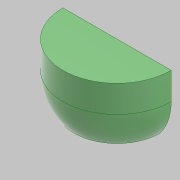
# Autodesk Inventor part: 본체
Saved by Autodesk Inventor 2020 (Build 240168000, 168)
## iProperties
Created: 2020-05-03
Part Number: 본체
Material: 일반
Document SubType Name: Modeling
Designer: sbahn
Density: 1 g/cm^3
Appearance: 매끄러움 - 짙은 산림 녹색
Author: sbahn
Autodesk Inventor part; units mm, degrees
(part 1 of 2)
ref_plane "XZ Plane" through (0, 0, 0) normal (0, 1, 0) x (-1, 0, 0)
ref_plane "XY Plane" through (0, 0, 0) normal (0, 0, 1) x (1, 0, 0)
sketch "스케치1" plane through (0, 0, 0) normal (0, 1, 0) x (-1, 0, 0)
  line L0 (-14.5321, -10.5819) -> (-29.968, -35.283)
  arc A0 (-38.4205, -39.9689) -> (-29.968, -35.283) centre (-38.422, -30) ccw
  line L1 (-38.4205, -39.9689) -> (-120.878, -39.9798)
  line L2 (-120.8795, 40) -> (-38.422, 40)
  arc A1 (-29.942, 35.3) -> (-38.422, 40) centre (-38.422, 30) ccw
  line L3 (-29.942, 35.3) -> (-14.5328, 10.583)
  line L4 (-18.7445, -7.95) -> (-34.182, -32.65)
  arc A2 (-38.422, -35) -> (-34.182, -32.65) centre (-38.422, -30) ccw
  line L5 (-38.422, -35) -> (-120.8795, -35)
  line L6 (-120.8795, 35) -> (-38.422, 35)
  arc A3 (-34.182, 32.65) -> (-38.422, 35) centre (-38.422, 30) ccw
  line L7 (-34.182, 32.65) -> (-18.7445, 7.95)
  line L8 (-133.9879, -34.9502) -> (-133.9879, -34.9502)
  line L9 (0, 0) -> (-214.2408, 0)
  line L10 (-97.3795, -37.5) -> (-100.3795, -37.5)
  line L11 (-104.8795, -3.3) -> (-104.8795, -27.5)
  line L12 (-66.878, -39.9727) -> (-66.8787, -35)
  line L13 (-62.878, -39.9722) -> (-62.8787, -35)
  line L14 (-64.8795, -35) -> (-64.8795, -34)
  line L15 (-80.8795, -35) -> (-80.8795, -34)
  line L16 (-78.8787, -35) -> (-78.878, -39.9743)
  line L17 (-59.8795, -39.9718) -> (-59.8795, -48)
  line L18 (-85.8795, -48) -> (-85.8795, -39.9752)
  line L19 (-67.8795, -39.9728) -> (-67.8795, -48)
  line L20 (-73.8795, -29) -> (-73.8795, -83)
  line L21 (-71.8795, -83) -> (-71.8795, -29)
  line L22 (-85.8795, -48) -> (-59.8795, -48)
  line L23 (-77.8795, -48) -> (-77.8795, -39.9741)
  line L24 (-87.7712, -44) -> (-71.8795, -44)
  line L25 (-85.8795, -45.5) -> (-77.8795, -45.5)
  line L26 (-85.8795, -42.5) -> (-77.8795, -42.5)
  line L27 (-77.8795, -42.5) -> (-76.2373, -44)
  line L28 (-76.2373, -44) -> (-77.8795, -45.5)
  line L29 (-72.8795, -48) -> (-55.3795, -48)
  line L30 (-90.3795, -53) -> (-90.3795, -48)
  line L31 (-127.8795, -53) -> (-127.8795, -89)
  line L32 (-127.8795, -89) -> (-17.8795, -89)
  line L33 (-17.8795, -89) -> (-17.8795, -53)
  line L34 (-17.8795, -53) -> (-127.8795, -53)
  line L35 (-126.8795, -54) -> (-18.8795, -54)
  line L36 (-18.8795, -54) -> (-18.8795, -88)
  line L37 (-18.8795, -88) -> (-126.8795, -88)
  line L38 (-126.8795, -88) -> (-126.8795, -54)
  line L39 (-55.3795, -59) -> (-90.3795, -59)
  line L40 (-90.3795, -54) -> (-90.3795, -59)
  line L41 (-71.8795, -48) -> (-71.8795, -59)
  line L42 (-73.8795, -48) -> (-73.8795, -59)
  line L43 (-85.8795, -48) -> (-90.3795, -48)
  line L44 (-88.1295, -46.2635) -> (-88.1295, -60.7681)
  line L45 (-57.6295, -46.0218) -> (-57.6295, -60.2242)
  line L46 (-87.1295, -49.1111) -> (-85.8795, -48)
  line L47 (-89.1295, -49.1111) -> (-90.3795, -48)
  line L48 (-89.1295, -49.1111) -> (-89.1295, -59)
  line L49 (-87.1295, -49.1111) -> (-87.1295, -59)
  line L50 (-87.1295, -49.1111) -> (-89.1295, -49.1111)
  line L51 (-55.3795, -53) -> (-55.3795, -48)
  line L52 (-55.3795, -54) -> (-55.3795, -59)
  line L53 (-58.6295, -49.1111) -> (-59.8795, -48)
  line L54 (-56.6295, -49.1111) -> (-55.3795, -48)
  line L55 (-56.6295, -49.1111) -> (-56.6295, -59)
  line L56 (-58.6295, -49.1111) -> (-58.6295, -59)
  line L57 (-58.6295, -49.1111) -> (-56.6295, -49.1111)
  line L58 (-8.3175, -71) -> (-138.1557, -71)
  line L59 (-90.3795, -94) -> (-78.8795, -94)
  line L60 (-66.8795, -94) -> (-55.3795, -94)
  line L61 (-90.3795, -89) -> (-90.3795, -94)
  line L62 (-55.3795, -83) -> (-90.3795, -83)
  line L63 (-90.3795, -88) -> (-90.3795, -83)
  line L64 (-71.8795, -92) -> (-71.8795, -83)
  line L65 (-73.8795, -92) -> (-73.8795, -83)
  line L66 (-88.1295, -95.7365) -> (-88.1295, -81.2319)
  line L67 (-57.6295, -95.9782) -> (-57.6295, -81.7758)
  line L68 (-87.1295, -92.8889) -> (-85.8795, -94)
  line L69 (-89.1295, -92.8889) -> (-90.3795, -94)
  line L70 (-89.1295, -92.8889) -> (-89.1295, -83)
  line L71 (-87.1295, -92.8889) -> (-87.1295, -83)
  line L72 (-87.1295, -92.8889) -> (-89.1295, -92.8889)
  line L73 (-55.3795, -89) -> (-55.3795, -94)
  line L74 (-55.3795, -88) -> (-55.3795, -83)
  line L75 (-58.6295, -92.8889) -> (-59.8795, -94)
  line L76 (-56.6295, -92.8889) -> (-55.3795, -94)
  line L77 (-56.6295, -92.8889) -> (-56.6295, -83)
  line L78 (-58.6295, -92.8889) -> (-58.6295, -83)
  line L79 (-58.6295, -92.8889) -> (-56.6295, -92.8889)
  line L80 (-74.8795, -71) -> (-70.8795, -71)
  line L81 (-71.8795, -83) -> (-71.8795, -59)
  line L82 (-73.8795, -59) -> (-73.8795, -83)
  line L83 (-72.8795, -59) -> (-64.8795, -59)
  line L84 (-64.8795, -59) -> (-70.8795, -71)
  line L85 (-72.8795, -59) -> (-80.8795, -59)
  line L86 (-80.8795, -59) -> (-74.8795, -71)
  line L87 (-72.8795, -83) -> (-80.8795, -83)
  line L88 (-80.8795, -83) -> (-74.8795, -71)
  line L89 (-72.8795, -83) -> (-64.8795, -83)
  line L90 (-64.8795, -83) -> (-70.8795, -71)
  line L91 (-66.8795, 40) -> (-66.8795, 35)
  line L92 (-62.8795, 40) -> (-62.8795, 35)
  line L93 (-64.8795, 35) -> (-64.8795, 34)
  line L94 (-80.8795, 35) -> (-80.8795, 34)
  line L95 (-78.8795, 35) -> (-78.8795, 40)
  line L96 (-59.8795, 40) -> (-59.8795, 48)
  line L97 (-85.8795, 48) -> (-85.8795, 40)
  line L98 (-67.8795, 40) -> (-67.8795, 48)
  line L99 (-73.8795, 29) -> (-73.8795, 48)
  line L100 (-71.8795, 48) -> (-71.8795, 29)
  line L101 (-85.8795, 48) -> (-59.8795, 48)
  line L102 (-77.8795, 48) -> (-77.8795, 40)
  line L103 (-87.7712, 44) -> (-71.8795, 44)
  line L104 (-85.8795, 45.5) -> (-77.8795, 45.5)
  line L105 (-85.8795, 42.5) -> (-77.8795, 42.5)
  line L106 (-77.8795, 42.5) -> (-76.2373, 44)
  line L107 (-76.2373, 44) -> (-77.8795, 45.5)
  line L108 (-72.8795, 48) -> (-55.3795, 48)
  line L109 (-90.3795, 53) -> (-90.3795, 48)
  line L110 (-127.8795, 53) -> (-127.8795, 89)
  line L111 (-127.8795, 89) -> (-17.8795, 89)
  line L112 (-17.8795, 89) -> (-17.8795, 53)
  line L113 (-17.8795, 53) -> (-127.8795, 53)
  line L114 (-126.8795, 54) -> (-18.8795, 54)
  line L115 (-18.8795, 54) -> (-18.8795, 88)
  line L116 (-18.8795, 88) -> (-126.8795, 88)
  line L117 (-126.8795, 88) -> (-126.8795, 54)
  line L118 (-55.3795, 59) -> (-90.3795, 59)
  line L119 (-90.3795, 54) -> (-90.3795, 59)
  line L120 (-71.8795, 48) -> (-71.8795, 59)
  line L121 (-73.8795, 48) -> (-73.8795, 59)
  line L122 (-85.8795, 48) -> (-90.3795, 48)
  line L123 (-88.1295, 46.2635) -> (-88.1295, 60.7681)
  line L124 (-57.6295, 46.0218) -> (-57.6295, 60.2242)
  line L125 (-87.1295, 49.1111) -> (-85.8795, 48)
  line L126 (-89.1295, 49.1111) -> (-90.3795, 48)
  line L127 (-89.1295, 49.1111) -> (-89.1295, 59)
  line L128 (-87.1295, 49.1111) -> (-87.1295, 59)
  line L129 (-87.1295, 49.1111) -> (-89.1295, 49.1111)
  line L130 (-55.3795, 53) -> (-55.3795, 48)
  line L131 (-55.3795, 54) -> (-55.3795, 59)
  line L132 (-58.6295, 49.1111) -> (-59.8795, 48)
  line L133 (-56.6295, 49.1111) -> (-55.3795, 48)
  line L134 (-56.6295, 49.1111) -> (-56.6295, 59)
  line L135 (-58.6295, 49.1111) -> (-58.6295, 59)
  line L136 (-58.6295, 49.1111) -> (-56.6295, 49.1111)
  line L137 (-8.3175, 71) -> (-138.1557, 71)
  line L138 (-90.3795, 94) -> (-78.8795, 94)
  line L139 (-66.8795, 94) -> (-55.3795, 94)
  line L140 (-55.3795, 94) -> (-55.3795, 89)
  line L141 (-90.3795, 89) -> (-90.3795, 94)
  line L142 (-55.3795, 88) -> (-55.3795, 83)
  line L143 (-55.3795, 83) -> (-90.3795, 83)
  line L144 (-90.3795, 88) -> (-90.3795, 83)
  line L145 (-71.8795, 92) -> (-71.8795, 48)
  line L146 (-73.8795, 92) -> (-73.8795, 48)
  line L147 (-88.1295, 95.7365) -> (-88.1295, 81.2319)
  line L148 (-57.6295, 95.9782) -> (-57.6295, 81.7758)
  line L149 (-87.1295, 92.8889) -> (-85.8795, 94)
  line L150 (-89.1295, 92.8889) -> (-90.3795, 94)
  line L151 (-89.1295, 92.8889) -> (-89.1295, 83)
  line L152 (-87.1295, 92.8889) -> (-87.1295, 83)
  line L153 (-87.1295, 92.8889) -> (-89.1295, 92.8889)
  line L154 (-58.6295, 92.8889) -> (-59.8795, 94)
  line L155 (-56.6295, 92.8889) -> (-55.3795, 94)
  line L156 (-56.6295, 92.8889) -> (-56.6295, 83)
  line L157 (-58.6295, 92.8889) -> (-58.6295, 83)
  line L158 (-58.6295, 92.8889) -> (-56.6295, 92.8889)
  line L159 (-74.8795, 71) -> (-70.8795, 71)
  line L160 (-71.8795, 83) -> (-71.8795, 59)
  line L161 (-73.8795, 59) -> (-73.8795, 83)
  line L162 (-72.8795, 59) -> (-64.8795, 59)
  line L163 (-64.8795, 59) -> (-70.8795, 71)
  line L164 (-72.8795, 59) -> (-80.8795, 59)
  line L165 (-80.8795, 59) -> (-74.8795, 71)
  line L166 (-72.8795, 83) -> (-80.8795, 83)
  line L167 (-80.8795, 83) -> (-74.8795, 71)
  line L168 (-72.8795, 83) -> (-64.8795, 83)
  line L169 (-64.8795, 83) -> (-70.8795, 71)
  line L170 (-72.8795, -104.0341) -> (-72.8795, 102.0223)
  line L171 (-85.8795, -28) -> (-85.8795, -35)
  line L172 (-87.8795, -29) -> (-87.8795, -34)
  line L173 (-88.3795, -29) -> (-88.3795, -34)
  line L174 (-83.3795, -29) -> (-83.3795, -34)
  line L175 (-59.8795, -28) -> (-59.8795, -35)
  line L176 (-57.8795, -29) -> (-57.8795, -34)
  line L177 (-62.3795, -29) -> (-62.3795, -34)
  line L178 (-57.8795, -34) -> (-113.8795, -34)
  line L179 (-57.8795, -29) -> (-113.8795, -29)
  line L180 (-111.8795, -28) -> (-111.8795, -35)
  line L181 (-113.8795, -29) -> (-113.8795, -34)
  line L182 (-109.3795, -29) -> (-109.3795, -34)
  line L183 (-98.8795, -45.3206) -> (-98.8795, 49.0244)
  line L184 (-82.8795, 35) -> (-82.8795, 40)
  line L185 (-100.8795, -27.5) -> (-100.8795, -28.3)
  line L186 (-100.8795, -28.3) -> (-96.8795, -28.3)
  line L187 (-96.8795, -28.3) -> (-96.8795, -27.5)
  line L188 (-100.3795, -38) -> (-97.3795, -38)
  line L189 (-109.7745, -27.5) -> (-87.8795, -27.5)
  line L190 (-97.3795, 37.5) -> (-100.3795, 37.5)
  line L191 (-104.8795, 3.3) -> (-104.8795, 27.5)
  line L192 (-111.8795, 28) -> (-111.8795, 35)
  line L193 (-113.8795, 29) -> (-113.8795, 34)
  line L194 (-109.3795, 29) -> (-109.3795, 34)
  line L195 (-100.8795, 27.5) -> (-100.8795, 28.3)
  line L196 (-100.8795, 28.3) -> (-96.8795, 28.3)
  line L197 (-96.8795, 28.3) -> (-96.8795, 27.5)
  line L198 (-100.3795, 38) -> (-100.3795, 27.5)
  line L199 (-100.3795, 38) -> (-97.3795, 38)
  line L200 (-97.3795, 38) -> (-97.3795, 27.5)
  line L201 (-109.8795, 27.5) -> (-87.8795, 27.5)
  line L202 (-87.8795, 27.5) -> (-87.8795, -27.5)
  line L203 (-109.8795, 27.5) -> (-109.8795, 9.2)
  line L204 (-109.7745, -9.2011) -> (-109.7745, -27.5)
  line L205 (-85.8795, 28) -> (-85.8795, 35)
  line L206 (-87.8795, 29) -> (-87.8795, 34)
  line L207 (-88.3795, 29) -> (-88.3795, 34)
  line L208 (-83.3795, 29) -> (-83.3795, 34)
  line L209 (-59.8795, 28) -> (-59.8795, 35)
  line L210 (-57.8795, 29) -> (-57.8795, 34)
  line L211 (-62.3795, 29) -> (-62.3795, 34)
  line L212 (-57.8795, 34) -> (-113.8795, 34)
  line L213 (-57.8795, 29) -> (-113.8795, 29)
  line L214 (-87.8795, -14.5) -> (-92.8795, -14.5)
  line L215 (-104.8795, -14.5) -> (-109.7745, -14.5)
  circle A4 centre (-90.3795, -14.5) radius 1.5
  circle A5 centre (-107.3795, -14.5) radius 1.5
  line L216 (-90.3795, -16.8389) -> (-90.3795, -12.0774)
  line L217 (-107.3795, -16.983) -> (-107.3795, -11.7622)
  line L218 (-87.8795, 14.5) -> (-92.8795, 14.5)
  line L219 (-104.8795, 14.5) -> (-109.8795, 14.5)
  circle A6 centre (-90.3795, 14.5) radius 1.5
  circle A7 centre (-107.3795, 14.5) radius 1.5
  line L220 (-90.3795, 16.8389) -> (-90.3795, 12.0774)
  line L221 (-107.3795, 16.983) -> (-107.3795, 11.7622)
  line L222 (-108.5248, -3.3) -> (-91.8795, -3.3)
  line L223 (-91.8795, -3.3) -> (-91.8795, 3.3)
  line L224 (-91.8795, 3.3) -> (-108.5248, 3.3)
  line L225 (-94.453, 3.3) -> (-94.453, 2.069)
  line L226 (-94.453, 2.069) -> (-94.1325, 2.069)
  line L227 (-94.1325, 2.069) -> (-94.1325, 3.3)
  line L228 (-103.306, 3.3) -> (-103.306, 2.069)
  line L229 (-103.306, 2.069) -> (-103.6265, 2.069)
  line L230 (-103.6265, 2.069) -> (-103.6265, 3.3)
  line L231 (-96.5487, 3.3) -> (-96.5487, 2.7093)
  line L232 (-96.5487, 2.7093) -> (-101.2104, 2.7093)
  line L233 (-101.2104, 3.3) -> (-101.2104, 2.7093)
  line L234 (-92.8795, 27.5) -> (-92.8795, 3.3)
  line L235 (-82.8787, -35) -> (-82.878, -39.9748)
  line L236 (-92.8795, -27.5) -> (-92.8795, -3.3)
  line L237 (-100.3795, -38) -> (-100.3795, -27.5)
  line L238 (-97.3795, -27.5) -> (-97.3795, -38)
  line L239 (-94.453, -3.3) -> (-94.453, -2.069)
  line L240 (-94.453, -2.069) -> (-94.1325, -2.069)
  line L241 (-94.1325, -2.069) -> (-94.1325, -3.3)
  line L242 (-103.306, -3.3) -> (-103.306, -2.069)
  line L243 (-103.306, -2.069) -> (-103.6265, -2.069)
  line L244 (-103.6265, -2.069) -> (-103.6265, -3.3)
  line L245 (-96.5487, -3.3) -> (-96.5487, -2.7093)
  line L246 (-96.5487, -2.7093) -> (-101.2104, -2.7093)
  line L247 (-101.2104, -3.3) -> (-101.2104, -2.7093)
  line L248 (-99.0407, 2.7093) -> (-99.0407, 2.0857)
  line L249 (-98.7184, 2.7093) -> (-98.7184, 2.0857)
  line L250 (-98.7184, 2.0857) -> (-99.0407, 2.0857)
  line L251 (-99.0407, -2.7093) -> (-99.0407, -2.0857)
  line L252 (-98.7184, -2.7093) -> (-98.7184, -2.0857)
  line L253 (-98.7184, -2.0857) -> (-99.0407, -2.0857)
  line L254 (-41.6795, -6) -> (-65.8795, -6)
  line L255 (-65.8795, -2) -> (-66.6795, -2)
  line L256 (-66.6795, -2) -> (-66.6795, 2)
  line L257 (-66.6795, 2) -> (-65.8795, 2)
  line L258 (-75.8795, -1.5) -> (-66.6795, -1.5)
  line L259 (-75.8795, 1.5) -> (-66.6795, 1.5)
  line L260 (-41.6795, 4.4265) -> (-40.4485, 4.4265)
  line L261 (-40.4485, 4.4265) -> (-40.4485, 4.747)
  line L262 (-40.4485, 4.747) -> (-41.6795, 4.747)
  line L263 (-41.6795, -4.4265) -> (-40.4485, -4.4265)
  line L264 (-40.4485, -4.4265) -> (-40.4485, -4.747)
  line L265 (-40.4485, -4.747) -> (-41.6795, -4.747)
  line L266 (-41.6795, 2.3309) -> (-41.0888, 2.3309)
  line L267 (-41.0888, 2.3309) -> (-41.0888, -2.3309)
  line L268 (-41.6795, -2.3309) -> (-41.0888, -2.3309)
  line L269 (-65.8795, 6) -> (-41.6795, 6)
  line L270 (-41.0888, -0.1611) -> (-40.4653, -0.1611)
  line L271 (-41.0888, 0.1611) -> (-40.4653, 0.1611)
  line L272 (-40.4653, 0.1611) -> (-40.4653, -0.1611)
  line L273 (-92.8795, -18.5) -> (-104.8795, -18.5)
  line L274 (-104.8795, 18.5) -> (-92.8795, 18.5)
  line L275 (-56.8795, 6) -> (-56.8795, -6)
  line L276 (-69.8795, 6.5) -> (-69.8795, -6.5)
  line L277 (-69.8795, -6.5) -> (-75.8795, -6.5)
  line L278 (-75.8795, -6.5) -> (-75.8795, 6.5)
  line L279 (-75.8795, 6.5) -> (-69.8795, 6.5)
  line L280 (-69.8795, 5) -> (-66.8795, 5)
  line L281 (-66.8795, 5) -> (-66.8795, -5)
  line L282 (-66.8795, -5) -> (-69.8795, -5)
  line L283 (-72.3795, 4.5493) -> (-72.3795, 1.5)
  line L284 (-72.3795, -1.5) -> (-72.3795, -4.5493)
  line L285 (-73.3795, 4.5493) -> (-73.3795, 1.5)
  line L286 (-73.3795, -1.5) -> (-73.3795, -4.5493)
  arc A8 (-70.3795, -6.5) -> (-75.3795, -6.5) centre (-72.8795, -7.0625) ccw
  arc A9 (-75.3795, 6.5) -> (-70.3795, 6.5) centre (-72.8795, 7.0625) ccw
  arc A10 (-14.5321, -10.5819) -> (-14.5328, 10.583) centre (-31.4645, 0) ccw
  arc A11 (-14.9564, -10.3174) -> (-14.9567, 10.3178) centre (-31.4645, 0) ccw
  arc A12 (-18.7445, -7.95) -> (-18.7445, 7.95) centre (-31.4645, 0) ccw
  arc A13 (-194.777, 7.282) -> (-194.7731, -7.2802) centre (-191.4606, 0.0018) ccw
  arc A14 (-120.8795, 40) -> (-125.0298, 39.0981) centre (-120.8795, 30) ccw
  arc A15 (-120.8795, 35) -> (-122.9546, 34.5491) centre (-120.8795, 30) ccw
  line L287 (-194.777, 7.282) -> (-125.0298, 39.0981)
  line L288 (-125.0298, 39.0981) -> (-194.7847, 7.2785)
  line L289 (-122.9546, 34.5491) -> (-178.5248, 9.2)
  arc A16 (-125.0008, -39.0412) -> (-120.878, -39.9798) centre (-120.7742, -30.0006) ccw
  arc A17 (-122.8496, -34.5501) -> (-120.8795, -35) centre (-120.7742, -30.0006) ccw
  line L290 (-194.7731, -7.2802) -> (-125.0008, -39.0412)
  line L291 (-125.0008, -39.0412) -> (-194.777, -7.2785)
  line L292 (-122.8496, -34.5501) -> (-178.4197, -9.2011)
  line L293 (-178.5248, 9.2) -> (-178.4197, -9.2011)
  line L294 (-180.4251, -9.2011) -> (-108.5248, -9.2011)
  line L295 (-108.5248, -9.2011) -> (-108.5248, 9.2)
  line L296 (-108.5248, 9.2) -> (-180.4251, 9.2)
  line L297 (-180.4251, -9.2011) -> (-180.4251, 9.2)
  line L298 (-41.6795, -10.5) -> (-65.8795, -10.5)
  line L299 (-65.8795, -10.5) -> (-65.8795, 10.5)
  line L300 (-65.8795, 10.5) -> (-41.6795, 10.5)
  line L301 (-41.6795, 10.5) -> (-41.6795, -10.5)
  circle A18 centre (-46.1795, -8.25) radius 1.5
  circle A19 centre (-61.3795, -8.25) radius 1.5
  circle A20 centre (-61.3795, 8.25) radius 1.5
  circle A21 centre (-46.1795, 8.25) radius 1.5
  line L302 (-43.3628, -8.25) -> (-63.8935, -8.25)
  line L303 (-43.3124, 8.25) -> (-63.843, 8.25)
  line L304 (-61.3795, -10.7982) -> (-61.3795, -5.405)
  line L305 (-46.1795, -11.0295) -> (-46.1795, -5.362)
  line L306 (-46.1795, 5.2057) -> (-46.1795, 11.2164)
  line L307 (-61.3795, 5.1324) -> (-61.3795, 11.1798)
  line L308 (-14.9564, -10.3174) -> (-14.3696, -10.3174)
  line L309 (-14.9567, 10.3178) -> (-14.3703, 10.3185)
  line L310 (-12.6257, -4.9057) -> (-17.7189, -4.9058)
  line L311 (-17.7189, -3.4079) -> (-20.9821, -3.4079)
  line L312 (-20.9821, -2.096) -> (-23.4937, -2.096)
  line L313 (-23.4937, -7.0903) -> (-24.761, -7.0903)
  line L314 (-12.6259, 4.9063) -> (-17.719, 4.9063)
  line L315 (-17.719, 4.9063) -> (-17.7189, -4.9058)
  line L316 (-17.719, 3.4079) -> (-20.9821, 3.4079)
  line L317 (-20.9821, 3.4079) -> (-20.9821, -3.4079)
  line L318 (-20.9821, 2.096) -> (-23.4937, 2.096)
  line L319 (-23.4937, -7.0903) -> (-23.4937, 7.0903)
  line L320 (-23.4937, 7.0903) -> (-24.761, 7.0903)
  line L321 (-24.761, 7.0903) -> (-24.761, -7.0903)
  line L322 (-12.6257, -4.9057) -> (-12.6259, 4.9063)
  line L323 (-66.8795, -94) -> (-66.8795, -92)
  line L324 (-66.8795, -92) -> (-78.8795, -92)
  line L325 (-78.8795, -92) -> (-78.8795, -94)
  line L326 (-72.8795, -92) -> (-67.8795, -92)
  line L327 (-67.8795, -92) -> (-67.8795, -95)
  line L328 (-67.8795, -95) -> (-77.8795, -95)
  line L329 (-77.8795, -95) -> (-77.8795, -92)
  line L330 (-66.8795, 94) -> (-66.8795, 92)
  line L331 (-66.8795, 92) -> (-78.8795, 92)
  line L332 (-78.8795, 92) -> (-78.8795, 94)
  line L333 (-67.8795, 92) -> (-67.8795, 95)
  line L334 (-67.8795, 95) -> (-77.8795, 95)
  line L335 (-77.8795, 95) -> (-77.8795, 92)
  line L336 (-61.6632, -40) -> (-59.8795, -41.7837)
  line L337 (-63.9083, -40) -> (-59.8795, -44.0288)
  line L338 (-66.1533, -40) -> (-59.8795, -46.2738)
  line L339 (-67.8795, -40.5189) -> (-60.3984, -48)
  line L340 (-67.8795, -42.764) -> (-62.6435, -48)
  line L341 (-67.8795, -45.009) -> (-64.8885, -48)
  line L342 (-67.8795, -47.2541) -> (-67.1336, -48)
  line L343 (-79.6237, -40) -> (-77.8795, -41.7442)
  line L344 (-81.8688, -40) -> (-79.3688, -42.5)
  line L345 (-84.1139, -40) -> (-81.6139, -42.5)
  line L346 (-78.6139, -45.5) -> (-77.8795, -46.2343)
  line L347 (-85.8795, -40.4794) -> (-83.8589, -42.5)
  line L348 (-80.8589, -45.5) -> (-78.3589, -48)
  line L349 (-83.104, -45.5) -> (-80.604, -48)
  line L350 (-85.3491, -45.5) -> (-82.8491, -48)
  line L351 (-85.8795, -47.2146) -> (-85.0941, -48)
  line L352 (-69.813, 48) -> (-67.8795, 46.0665)
  line L353 (-71.8795, 47.8214) -> (-67.8795, 43.8214)
  line L354 (-74.3032, 48) -> (-73.8795, 47.5763)
  line L355 (-71.8795, 45.5763) -> (-67.8795, 41.5763)
  line L356 (-76.5482, 48) -> (-73.8795, 45.3313)
  line L357 (-62.5482, 34) -> (-62.3795, 33.8313)
  line L358 (-71.8795, 43.3313) -> (-68.5482, 40)
  line L359 (-68.5482, 40) -> (-66.8795, 38.3313)
  line L360 (-77.8795, 47.0862) -> (-74.7933, 44)
  line L361 (-64.7933, 34) -> (-62.3795, 31.5862)
  line L362 (-74.7933, 44) -> (-73.8795, 43.0862)
  line L363 (-65.7933, 35) -> (-64.8795, 34.0862)
  line L364 (-71.8795, 41.0862) -> (-70.7933, 40)
  line L365 (-70.7933, 40) -> (-66.8795, 36.0862)
  line L366 (-76.656, 43.6176) -> (-73.8795, 40.8412)
  line L367 (-67.0384, 34) -> (-62.3795, 29.3412)
  line L368 (-71.8795, 38.8412) -> (-68.0384, 35)
  line L369 (-68.0384, 35) -> (-67.0384, 34)
  line L370 (-77.8293, 42.5459) -> (-75.2834, 40)
  line L371 (-69.2834, 34) -> (-64.2834, 29)
  line L372 (-75.2834, 40) -> (-73.8795, 38.5961)
  line L373 (-70.2834, 35) -> (-69.2834, 34)
  line L374 (-71.8795, 36.5961) -> (-70.2834, 35)
  line L375 (-77.8795, 40.351) -> (-77.5285, 40)
  line L376 (-71.5285, 34) -> (-66.5285, 29)
  line L377 (-77.5285, 40) -> (-73.8795, 36.351)
  line L378 (-71.8795, 34.351) -> (-71.5285, 34)
  line L379 (-78.8795, 39.106) -> (-74.7736, 35)
  line L380 (-71.8795, 32.106) -> (-68.7736, 29)
  line L381 (-74.7736, 35) -> (-73.8795, 34.106)
  line L382 (-78.8795, 36.8609) -> (-77.0186, 35)
  line L383 (-71.8795, 29.8609) -> (-71.0186, 29)
  line L384 (-77.0186, 35) -> (-76.0186, 34)
  line L385 (-76.0186, 34) -> (-73.8795, 31.8609)
  line L386 (-79.2637, 35) -> (-78.2637, 34)
  line L387 (-78.2637, 34) -> (-73.8795, 29.6158)
  line L388 (-80.8795, 34.3708) -> (-80.5088, 34)
  line L389 (-80.5088, 34) -> (-75.5088, 29)
  line L390 (-82.7538, 34) -> (-77.7538, 29)
  line L391 (-83.3795, 32.3806) -> (-79.9989, 29)
  line L392 (-83.3795, 30.1356) -> (-82.2439, 29)
  line L393 (-62.8795, -39.3331) -> (-63.5464, -40)
  line L394 (-62.8795, -37.088) -> (-65.7915, -40)
  line L395 (-63.0366, -35) -> (-66.8795, -38.843)
  line L396 (-65.2816, -35) -> (-66.8795, -36.5979)
  line L397 (-78.8795, -39.6176) -> (-79.2619, -40)
  line L398 (-78.8795, -37.3726) -> (-81.5069, -40)
  line L399 (-78.8795, -35.1275) -> (-82.8795, -39.1275)
  line L400 (-80.9971, -35) -> (-82.8795, -36.8825)
  line L401 (-62.41, -29) -> (-62.3795, -29.0305)
  line L402 (-64.6551, -29) -> (-62.3795, -31.2756)
  line L403 (-66.9002, -29) -> (-62.3795, -33.5206)
  line L404 (-69.1452, -29) -> (-64.1452, -34)
  line L405 (-71.3903, -29) -> (-66.3903, -34)
  line L406 (-66.3903, -34) -> (-65.3903, -35)
  line L407 (-71.8795, -30.7558) -> (-68.6354, -34)
  line L408 (-67.6354, -35) -> (-66.8795, -35.7558)
  line L409 (-68.6354, -34) -> (-67.6354, -35)
  line L410 (-75.8804, -29) -> (-73.8795, -31.0009)
  line L411 (-69.8804, -35) -> (-66.8795, -38.0009)
  line L412 (-71.8795, -33.0009) -> (-70.8804, -34)
  line L413 (-70.8804, -34) -> (-69.8804, -35)
  line L414 (-78.1255, -29) -> (-73.8795, -33.246)
  line L415 (-71.8795, -35.246) -> (-67.1255, -40)
  line L416 (-80.3705, -29) -> (-75.3705, -34)
  line L417 (-69.3705, -40) -> (-67.8795, -41.491)
  line L418 (-75.3705, -34) -> (-74.3705, -35)
  line L419 (-71.8795, -37.491) -> (-69.3705, -40)
  line L420 (-74.3705, -35) -> (-73.8795, -35.491)
  line L421 (-82.6156, -29) -> (-77.6156, -34)
  line L422 (-71.6156, -40) -> (-67.8795, -43.7361)
  line L423 (-77.6156, -34) -> (-76.6156, -35)
  line L424 (-71.8795, -39.7361) -> (-71.6156, -40)
  line L425 (-76.6156, -35) -> (-73.8795, -37.7361)
  line L426 (-83.3795, -30.4811) -> (-79.8607, -34)
  line L427 (-71.8795, -41.9811) -> (-67.8795, -45.9811)
  line L428 (-79.8607, -34) -> (-78.8607, -35)
  line L429 (-78.8607, -35) -> (-73.8795, -39.9811)
  line L430 (-83.3795, -32.7262) -> (-82.1057, -34)
  line L431 (-71.8795, -44.2262) -> (-68.1057, -48)
  line L432 (-78.8795, -37.2262) -> (-76.1057, -40)
  line L433 (-76.1057, -40) -> (-73.8795, -42.2262)
  line L434 (-78.8795, -39.4713) -> (-78.3508, -40)
  line L435 (-71.8795, -46.4713) -> (-70.3508, -48)
  line L436 (-77.8795, -40.4713) -> (-74.3508, -44)
  line L437 (-74.3508, -44) -> (-73.8795, -44.4713)
  line L438 (-76.4247, -44.1712) -> (-73.8795, -46.7163)
  line L439 (-77.598, -45.2429) -> (-74.8409, -48)
  line L440 (-77.8795, -47.2065) -> (-77.086, -48)
  line L441 (-56.6295, -54.014) -> (-55.3795, -55.264)
  line L442 (-58.8885, -54) -> (-58.6295, -54.259)
  line L443 (-56.6295, -56.259) -> (-55.3795, -57.509)
  line L444 (-61.1336, -54) -> (-58.6295, -56.5041)
  line L445 (-56.6295, -58.5041) -> (-56.1336, -59)
  line L446 (-63.3787, -54) -> (-58.6295, -58.7491)
  line L447 (-65.6237, -54) -> (-60.6237, -59)
  line L448 (-67.8688, -54) -> (-62.8688, -59)
  line L449 (-70.1139, -54) -> (-65.1139, -59)
  line L450 (-71.8795, -54.4794) -> (-67.3589, -59)
  line L451 (-74.604, -54) -> (-73.8795, -54.7245)
  line L452 (-71.8795, -56.7245) -> (-69.604, -59)
  line L453 (-76.8491, -54) -> (-73.8795, -56.9695)
  line L454 (-71.8795, -58.9695) -> (-71.8491, -59)
  line L455 (-79.0941, -54) -> (-74.0941, -59)
  line L456 (-81.3392, -54) -> (-76.3392, -59)
  line L457 (-83.5842, -54) -> (-78.5842, -59)
  line L458 (-85.8293, -54) -> (-80.8293, -59)
  line L459 (-87.1295, -54.9448) -> (-83.0744, -59)
  line L460 (-90.3194, -54) -> (-89.1295, -55.1899)
  line L461 (-87.1295, -57.1899) -> (-85.3194, -59)
  line L462 (-90.3795, -56.185) -> (-89.1295, -57.435)
  line L463 (-90.3795, -58.43) -> (-89.8096, -59)
  line L464 (-55.3795, -87.9597) -> (-55.4198, -88)
  line L465 (-55.3795, -85.7146) -> (-56.6295, -86.9646)
  line L466 (-55.3795, -83.4696) -> (-56.6295, -84.7196)
  line L467 (-58.6295, -86.7196) -> (-59.91, -88)
  line L468 (-58.6295, -84.4745) -> (-62.155, -88)
  line L469 (-59.4001, -83) -> (-64.4001, -88)
  line L470 (-61.6451, -83) -> (-66.6451, -88)
  line L471 (-63.8902, -83) -> (-68.8902, -88)
  line L472 (-66.1353, -83) -> (-71.1353, -88)
  line L473 (-68.3803, -83) -> (-71.8795, -86.4992)
  line L474 (-70.6254, -83) -> (-71.8795, -84.2541)
  line L475 (-73.8795, -86.2541) -> (-75.6254, -88)
  line L476 (-73.8795, -84.0091) -> (-77.8705, -88)
  line L477 (-75.1155, -83) -> (-80.1155, -88)
  line L478 (-77.3606, -83) -> (-82.3606, -88)
  line L479 (-79.6057, -83) -> (-84.6057, -88)
  line L480 (-81.8507, -83) -> (-86.8507, -88)
  line L481 (-84.0958, -83) -> (-87.1295, -86.0337)
  line L482 (-86.3409, -83) -> (-87.1295, -83.7887)
  line L483 (-89.1295, -85.7887) -> (-90.3795, -87.0387)
  line L484 (-89.1295, -83.5436) -> (-90.3795, -84.7936)
  line L485 (-62.1057, 48) -> (-59.8795, 45.7738)
  line L486 (-64.3508, 48) -> (-59.8795, 43.5287)
  line L487 (-66.5959, 48) -> (-59.8795, 41.2837)
  line L488 (-67.8795, 47.0386) -> (-60.8409, 40)
  line L489 (-67.8795, 44.7935) -> (-63.086, 40)
  line L490 (-67.8795, 42.5485) -> (-65.331, 40)
  line L491 (-67.8795, 40.3034) -> (-67.5761, 40)
  line L492 (-80.0662, 48) -> (-77.8795, 45.8133)
  line L493 (-82.3113, 48) -> (-79.8113, 45.5)
  line L494 (-84.5564, 48) -> (-82.0564, 45.5)
  line L495 (-79.0564, 42.5) -> (-77.8795, 41.3232)
  line L496 (-85.8795, 47.0781) -> (-84.3014, 45.5)
  line L497 (-81.3014, 42.5) -> (-78.8014, 40)
  line L498 (-83.5465, 42.5) -> (-81.0465, 40)
  line L499 (-85.7916, 42.5) -> (-83.2916, 40)
  line L500 (-85.8795, 40.3429) -> (-85.5366, 40)
  line L501 (-62.8795, 36.9991) -> (-64.8786, 35)
  line L502 (-62.8795, 39.2441) -> (-66.8795, 35.2441)
  line L503 (-64.3687, 40) -> (-66.8795, 37.4892)
  line L504 (-66.6138, 40) -> (-66.8795, 39.7343)
  line L505 (-78.8795, 36.7145) -> (-80.5941, 35)
  line L506 (-78.8795, 38.9596) -> (-82.8391, 35)
  line L507 (-80.0842, 40) -> (-82.8795, 37.2047)
  line L508 (-82.3292, 40) -> (-82.8795, 39.4497)
  line L509 (-56.6295, 58.2393) -> (-55.3795, 56.9893)
  line L510 (-59.6353, 59) -> (-58.6295, 57.9942)
  line L511 (-56.6295, 55.9942) -> (-55.3795, 54.7442)
  line L512 (-61.8804, 59) -> (-58.6295, 55.7491)
  line L513 (-64.1255, 59) -> (-59.1255, 54)
  line L514 (-66.3705, 59) -> (-61.3705, 54)
  line L515 (-68.6156, 59) -> (-63.6156, 54)
  line L516 (-70.8607, 59) -> (-65.8607, 54)
  line L517 (-71.8795, 57.7738) -> (-68.1057, 54)
  line L518 (-75.3508, 59) -> (-73.8795, 57.5287)
  line L519 (-71.8795, 55.5287) -> (-70.3508, 54)
  line L520 (-77.5959, 59) -> (-73.8795, 55.2837)
  line L521 (-79.8409, 59) -> (-74.8409, 54)
  line L522 (-82.086, 59) -> (-77.086, 54)
  line L523 (-84.331, 59) -> (-79.331, 54)
  line L524 (-86.5761, 59) -> (-81.5761, 54)
  line L525 (-87.1295, 57.3084) -> (-83.8212, 54)
  line L526 (-90.3795, 58.3133) -> (-89.1295, 57.0633)
  line L527 (-87.1295, 55.0633) -> (-86.0662, 54)
  line L528 (-90.3795, 56.0682) -> (-89.1295, 54.8182)
  line L529 (-55.3795, 84.9102) -> (-56.6295, 83.6602)
  line L530 (-55.3795, 87.1553) -> (-56.6295, 85.9053)
  line L531 (-58.6295, 83.9053) -> (-59.5348, 83)
  line L532 (-58.6295, 86.1504) -> (-61.7799, 83)
  line L533 (-59.025, 88) -> (-64.025, 83)
  line L534 (-61.27, 88) -> (-66.27, 83)
  line L535 (-63.5151, 88) -> (-68.5151, 83)
  line L536 (-65.7601, 88) -> (-70.7601, 83)
  line L537 (-68.0052, 88) -> (-71.8795, 84.1257)
  line L538 (-70.2503, 88) -> (-71.8795, 86.3707)
  line L539 (-73.8795, 84.3707) -> (-75.2503, 83)
  line L540 (-73.8795, 86.6158) -> (-77.4953, 83)
  line L541 (-74.7404, 88) -> (-79.7404, 83)
  line L542 (-76.9855, 88) -> (-81.9855, 83)
  line L543 (-79.2305, 88) -> (-84.2305, 83)
  line L544 (-81.4756, 88) -> (-86.4756, 83)
  line L545 (-83.7207, 88) -> (-87.1295, 84.5911)
  line L546 (-85.9657, 88) -> (-87.1295, 86.8362)
  line L547 (-89.1295, 84.8362) -> (-90.3795, 83.5862)
  line L548 (-89.1295, 87.0813) -> (-90.3795, 85.8313)
  line L549 (-50.9223, 0) -> (-50.9223, 123.6816)
  point P0 (-118.1661, -2.2051)
  constraints: 1068 end point, 145 point on line, 38 point on circle, 22 centre point, 3 midpoint, 1 vertical, 178 other
sketch "스케치2" plane through (0, 0, 0) normal (0, 1, 0) x (-1, 0, 0)
  line L0 (0, 0) -> (-236.664, 0) construction
  line L1 (-14.5321, -10.5819) -> (-29.968, -35.283) projected
  arc A0 (-38.4205, -39.9689) -> (-29.968, -35.283) centre (-38.422, -30) ccw projected
  line L2 (-38.4205, -39.9689) -> (-120.878, -39.9798) projected
  arc A1 (-125.0008, -39.0412) -> (-120.878, -39.9798) centre (-120.7742, -30.0006) ccw projected
  line L3 (-194.7731, -7.2802) -> (-125.0008, -39.0412) projected
  arc A2 (-194.777, 7.282) -> (-194.7731, -7.2802) centre (-191.4606, 0.0018) ccw projected
  line L4 (-194.777, 7.282) -> (-125.0298, 39.0981) projected
  arc A3 (-120.8795, 40) -> (-125.0298, 39.0981) centre (-120.8795, 30) ccw projected
  line L5 (-120.8795, 40) -> (-38.422, 40) projected
  arc A4 (-29.942, 35.3) -> (-38.422, 40) centre (-38.422, 30) ccw projected
  line L6 (-29.942, 35.3) -> (-14.5328, 10.583) projected
  arc A5 (-14.5321, -10.5819) -> (-14.5328, 10.583) centre (-31.4645, 0) ccw projected
  constraints: 2 end point, 1 horizontal
extrude "돌출1" add sketch "스케치2" along normal blind 45
delete faces "면 삭제1" heal yes whole lump no faces at (123.2348, 30, 39.7187) (121.3511, 30, -39.9637) (33.2971, 30, -38.5507) (33.282, 30, 38.5779) (13.7923, 30, 9.2938) (197.2446, 30, -5.5251)
sketch "스케치3" plane through (0, 0, 0) normal (0, 0, 1) x (1, 0, 0)
  line L0 (7.9273, 45) -> (7.9273, 0) projected
  line L1 (210.7534, 45) -> (210.7534, 0) projected
  line L2 (7.9273, 45) -> (210.7534, 45)
  line L3 (123.0526, 0) -> (210.7534, 0) projected
  line L4 (7.9273, 0) -> (210.7534, 0)
  line L5 (7.9273, 0) -> (7.9273, 5)
  line L6 (7.9273, 0) -> (77.9273, 0)
  line L7 (122.9382, 0) -> (32.8959, 0) projected
  line L8 (77.9273, 0) -> (7.9273, 5)
  line L9 (210.7534, 0) -> (122.9382, 0) projected
  line L10 (210.7534, 0) -> (210.7534, 25)
  line L11 (210.7534, 45) -> (122.9382, 45) projected
  line L12 (210.7534, 45) -> (122.9382, 45)
  line L13 (122.9382, 45) -> (210.7534, 25)
  line L14 (7.9273, 45) -> (7.9273, 32)
  line L15 (7.9273, 45) -> (47.9273, 45)
  line L16 (47.9273, 45) -> (7.9273, 32)
  line L17 (210.7534, 0) -> (210.7534, 3)
  line L18 (210.7534, 0) -> (176.7534, 0)
  line L19 (176.7534, 0) -> (210.7534, 3)
  point P0 (0, 0)
  dimension "d5" = 5
  dimension "d6" = 70
  dimension "d7" = 25
  dimension "d8" = 13
  dimension "d9" = 40
  dimension "d14" = 3
  dimension "d15" = 34
  constraints: 28 end point, 7 point on line, 2 horizontal, 1 collinear
  measures "d5" distance of L0.end L5.end
  measures "d6" distance of L0.end L6.end
  measures "d7" distance of L1.end L10.end
  measures "d8" distance of L0.start L14.end
  measures "d9" distance of L0.start L15.end
  measures "d14" distance of L1.end L17.end
  measures "d15" distance of L1.end L18.end
extrude "돌출2" cut sketch "스케치3" along normal mid plane 123.75 contours L2 L16 L0 | L8 L4 L0 | L2 L1 L13
fillet "모깎기1" radius 20 1 edges at (7.9273, 18.5, -0.0126)
fillet "모깎기2" radius 8 1 edges at (210.7534, 12.5, -0.0059)
shell "쉘1" thickness 5 removed faces 0
sketch "스케치5" plane through (121.854, 5, -34.9799) normal (0.0001319, 0, 1) x (1, 0, -0.0001319)
  ellipse E0 centre (-49.3506, 17.5) end of major axis (-39.3506, 17.5) minor radius 10 projected
  line L0 (-49.3506, 17.5) -> (-23.3506, 17.5)
  circle A0 centre (-23.3506, 17.5) radius 1.7
  point P0 (-121.8586, -5)
  dimension "d23" = 26
  dimension "d24" = 3.4
  constraints: 2 end point, 1 centre point, 1 coincident, 1 horizontal
  measures "d23" distance of L0.start L0.end
  measures "d24" diameter of A0
extrude "돌출4" cut sketch "스케치5" against normal blind 3 contours A0
mirror "미러1" about plane through (0, 0, 0) normal (0, 0, 1) of "돌출4"
sketch "스케치8" plane through (78.1056, 5, 35) normal (0, 1, 0) x (1, 0, 0)
  line L0 (22.0974, 72.9771) -> (18.6974, 72.9766) projected
  line L1 (22.0974, -2.9771) -> (18.6974, -2.9766) projected
  line L2 (20.3974, -2.9768) -> (20.3974, 72.9768)
  line L3 (9.3974, 62.5) -> (9.3974, 7.5)
  line L4 (9.3974, 7.5) -> (31.3974, 7.5)
  line L5 (31.3974, 7.5) -> (31.3974, 62.5)
  line L6 (31.3974, 62.5) -> (9.3974, 62.5)
  line L7 (9.3974, 62.5) -> (31.3974, 7.5) construction
  line L8 (9.3974, 7.5) -> (31.3974, 62.5) construction
  line L9 (20.3974, 35) -> (39.7063, 35) construction
  point P0 (-78.1056, 35)
  point P1 (20.3974, 35)
  dimension "d41" = 55
  dimension "d42" = 22
  constraints: 16 end point, 5 midpoint, 2 parallel, 1 horizontal, 1 perpendicular, 1 vertical
  measures "d41" distance of L3.start L3.end
  measures "d42" distance of L4.end L3.end
extrude "돌출6" add sketch "스케치8" along normal blind 17.5
sketch "스케치11" plane through (78.1056, 22.5, 35) normal (0, 1, 0) x (1, 0, 0)
  line L0 (31.3974, 7.5) -> (9.3974, 7.5)
  line L1 (9.3974, 7.5) -> (9.3974, 62.5)
  line L2 (9.3974, 62.5) -> (31.3974, 62.5)
  line L3 (31.3974, 62.5) -> (31.3974, 7.5)
  line L4 (11.8974, 49.5) -> (28.8974, 49.5)
  line L5 (28.8974, 49.5) -> (28.8974, 20.5)
  line L6 (28.8974, 20.5) -> (11.8974, 20.5)
  line L7 (11.8974, 20.5) -> (11.8974, 49.5)
  line L8 (11.8974, 35) -> (28.8974, 35) construction
  line L9 (20.3974, 49.5) -> (20.3974, 20.5) construction
  line L10 (9.3974, 35) -> (31.3974, 35) construction
  line L11 (20.3974, 35) -> (20.3974, 39.4317) construction
  point P0 (-78.1056, 35)
  point P1 (20.3974, 35)
  dimension "d52" = 17
  dimension "d53" = 29
  constraints: 24 end point, 8 midpoint, 5 coincident, 4 parallel, 2 horizontal, 2 perpendicular, 1 vertical
  measures "d52" distance of L5.end L6.end
  measures "d53" distance of L4.end L5.end
hole "구멍1" at (90.003, 22.5, -14.5) at (90.003, 22.5, 14.5) at (107.003, 22.5, 14.5) at (107.003, 22.5, -14.5) direction (0, -1, 0) diameter 2.5 depth 5 tip angle 118
sketch "스케치31" plane through (77.9273, 0, 40) normal (0, 0, 1) x (1, 0, 0)
  ellipse E0 centre (20.5761, 22.5) end of major axis (20.5761, 20.8) minor radius 1.7 projected
  ellipse E1 centre (20.5757, 22.5) end of major axis (20.5757, 20.8) minor radius 1.7 projected
  line L0 (20.5757, 22.5) -> (-5.4243, 22.5)
  circle A0 centre (-5.4243, 22.5) radius 10
  point P0 (-77.9273, 0)
  dimension "d122" = 26
  dimension "d123" = 20
  constraints: 2 end point, 1 centre point, 1 coincident, 1 horizontal, 2 other
  measures "d122" distance of L0.start L0.end
  measures "d123" diameter of A0
extrude "돌출16" cut sketch "스케치31" against normal blind 115.25 contours A0
sketch "스케치32" plane through (78.1056, 22.5, 35) normal (0, 1, 0) x (1, 0, 0)
  circle A0 centre (28.8974, 20.5) radius 1.25 projected
  circle A1 centre (11.8974, 49.5) radius 1.25 projected
  circle A2 centre (11.8974, 20.5) radius 1.25 projected
  circle A3 centre (28.8974, 49.5) radius 1.25 projected
  line L0 (31.3974, 7.5) -> (31.3974, 62.5) projected
  line L1 (31.3974, 62.5) -> (9.3974, 62.5) projected
  line L2 (9.3974, 62.5) -> (9.3974, 7.5) projected
  line L3 (9.3974, 7.5) -> (31.3974, 7.5) projected
  line L4 (20.3974, 62.5) -> (20.3974, 7.5)
  line L5 (14.3974, 7.5) -> (26.3974, 7.5)
  line L6 (26.3974, 7.5) -> (26.3974, 62.5)
  line L7 (26.3974, 62.5) -> (14.3974, 62.5)
  line L8 (14.3974, 62.5) -> (14.3974, 7.5)
  line L9 (14.3974, 7.5) -> (26.3974, 62.5) construction
  line L10 (26.3974, 7.5) -> (14.3974, 62.5) construction
  point P0 (-78.1056, 35)
  point P1 (20.3974, 35)
  point P2 (14.3974, 7.5)
  point P3 (26.3974, 7.5)
  dimension "d126" = 12
  constraints: 14 end point, 5 midpoint, 2 parallel, 1 horizontal, 1 perpendicular, 1 point on line
  measures "d126" distance of L7.end L6.end
extrude "돌출17" cut sketch "스케치32" along normal mid plane 10 contours L3 L4 L1 L6 | L3 L8 L1 L4
ref_plane "작업 평면4" through (78.1056, 16, 35) normal (0, 1, 0) x (1, 0, 0)
sketch "스케치16" plane through (78.1056, 5, 35) normal (0, 1, 0) x (1, 0, 0)
  line L0 (31.3974, 7.5) -> (31.3974, 62.5) projected
  line L1 (31.3974, 35) -> (155.4849, 35)
  line L2 (31.3974, 46.5) -> (102.3974, 46.5)
  line L3 (102.3974, 46.5) -> (102.3974, 23.5)
  line L4 (102.3974, 23.5) -> (31.3974, 23.5)
  line L5 (31.3974, 23.5) -> (31.3974, 46.5)
  line L6 (31.3974, 35) -> (102.3974, 35) construction
  line L7 (66.8974, 46.5) -> (66.8974, 23.5) construction
  line L8 (257.4456, 35) -> (-134.0308, 35) projected
  point P0 (-78.1056, 35)
  point P1 (66.8974, 35)
  point P2 (66.8974, 35)
  point P3 (31.3974, 23.5)
  point P4 (31.3974, 46.5)
  dimension "d71" = 71
  dimension "d72" = 23
  dimension "d73" = 0
  constraints: 14 end point, 7 midpoint, 2 horizontal, 2 parallel, 1 perpendicular, 1 point on line
  measures "d71" distance of L3.end L4.end
  measures "d72" distance of L2.end L3.end
  measures "d73" distance between parallel lines of L0 L5
extrude "돌출9" add sketch "스케치16" along normal blind 15
sketch "스케치15" plane through (78.1056, 16, 35) normal (0, 1, 0) x (1, 0, 0)
  circle A0 centre (28.8974, 20.5) radius 1.25 projected
  circle A1 centre (28.8974, 49.5) radius 1.25 projected
  line L0 (9.3974, 7.5) -> (14.3974, 7.5) projected
  line L1 (31.3974, 7.5) -> (31.3974, 62.5) projected
  line L2 (31.3974, 62.5) -> (26.3974, 62.5) projected
  line L3 (18.1626, 35) -> (128.06, 35)
  line L4 (29.8974, 44.3) -> (101.8974, 44.3)
  line L5 (101.8974, 44.3) -> (101.8974, 25.7)
  line L6 (101.8974, 25.7) -> (29.8974, 25.7)
  line L7 (29.8974, 25.7) -> (29.8974, 44.3)
  line L8 (29.8974, 35) -> (101.8974, 35) construction
  line L9 (65.8974, 44.3) -> (65.8974, 25.7) construction
  line L10 (274.8574, 35) -> (-136.9328, 35) projected
  line L11 (9.3974, 62.5) -> (9.3974, 7.5) projected
  line L12 (26.3974, 62.5) -> (26.3974, 7.5) projected
  line L13 (26.3974, 7.5) -> (31.3974, 7.5) projected
  line L14 (14.3974, 7.5) -> (14.3974, 62.5) projected
  line L15 (14.3974, 62.5) -> (9.3974, 62.5) projected
  point P0 (-78.1056, 35)
  point P1 (65.8974, 35)
  point P2 (101.8974, 35)
  point P3 (31.3974, 44.3)
  point P4 (31.3974, 35)
  dimension "d67" = 72
  dimension "d68" = 18.6
  dimension "d69" = 1.5
  constraints: 14 end point, 5 midpoint, 2 horizontal, 2 parallel, 1 perpendicular, 1 point on line
  measures "d67" distance of L5.end L6.end
  measures "d68" distance of L4.end L5.end
  measures "d69" distance between parallel lines of L7 L1
revolve "회전1" cut sketch "스케치15" angle 360 about axis through (96.2682, 16, 0) along (1, 0, 0) contours L1 L4 L5 L3
sketch "스케치17" plane through (109.503, 5, 27.5) normal (1, 0, 0) x (0, 0, -1)
  arc A0 (19.1042, 15) -> (35.8958, 15) centre (27.5, 11) ccw projected
  line L0 (18.2, 11) -> (36.8, 11)
  line L1 (36.8, 11) -> (18.2, 11)
  line L2 (18.2, 11) -> (18.2, 21.2919)
  line L3 (18.2, 21.2919) -> (36.8, 21.2919)
  line L4 (36.8, 21.2919) -> (36.8, 11)
  point P0 (27.5, -5)
  constraints: 10 end point, 2 horizontal, 2 parallel, 2 point on circle, 1 perpendicular
extrude "돌출10" cut sketch "스케치17" along normal blind 71
sketch "스케치18" plane through (87.503, 5, -27.5) normal (-1, 0, 0) x (0, 0, 1)
  line L0 (55, 17.5) -> (0, 17.5) construction
  line L1 (55, 0) -> (55, 17.5) construction
  line L2 (39, 0) -> (55, 0) projected
  line L3 (39, 0) -> (39, 15) construction
  line L4 (39, 15) -> (36.8, 15) construction
  line L5 (36.8, 15) -> (36.8, 11) construction
  arc A0 (18.2, 11) -> (36.8, 11) centre (27.5, 11) ccw construction
  line L6 (18.2, 11) -> (18.2, 15) construction
  line L7 (18.2, 15) -> (16, 15) construction
  line L8 (16, 15) -> (16, 0) construction
  line L9 (0, 0) -> (16, 0) projected
  line L10 (0, 0) -> (0, 17.5) construction
  line L11 (55, 12.5) -> (0, 12.5) projected
  line L12 (27.5, 17.5) -> (27.5, -5) construction
  line L13 (25, 10) -> (30, 10) construction
  line L14 (30, 10) -> (30, 5) construction
  line L15 (30, 5) -> (25, 5) construction
  line L16 (25, 5) -> (25, 10) construction
  line L17 (25, 10) -> (30, 5) construction
  line L18 (30, 10) -> (25, 5) construction
  line L19 (-122.0772, 17.5) -> (196.7247, 17.5) construction
  line L20 (6, 17.5) -> (6, -5) construction
  line L21 (55, 17.5) -> (0, 17.5) construction
  line L22 (49, 17.5) -> (49, -5) construction
  line L23 (3.5, 10) -> (13.5, 10)
  line L24 (13.5, 10) -> (13.5, 5)
  line L25 (13.5, 5) -> (3.5, 5)
  line L26 (3.5, 5) -> (3.5, 10)
  line L27 (41.5, 10) -> (51.5, 10)
  line L28 (51.5, 10) -> (51.5, 5)
  line L29 (51.5, 5) -> (41.5, 5)
  line L30 (41.5, 5) -> (41.5, 10)
  point P0 (27.5, 7.5)
  point P1 (6, 7.5)
  point P2 (49, 7.5)
  dimension "d78" = 5
  dimension "d79" = 5
  dimension "d80" = 2.5
  dimension "d81" = 43
  dimension "d82" = 21.5
  dimension "d84" = 5
  dimension "d86" = 5
  dimension "d188" = 2.5
  dimension "d189" = 10
  dimension "d190" = 2.5
  dimension "d191" = 10
  constraints: 34 end point, 6 parallel, 5 point on line, 3 horizontal, 3 midpoint, 3 perpendicular, 3 vertical
  measures "d78" distance of L14.end L15.end
  measures "d79" distance of L13.end L14.end
  measures "d80" distance between parallel lines of L11 L13
  measures "d81" distance between parallel lines of L20 L22
  measures "d82" distance between parallel lines of L12 L22
  measures "d84" distance of L23.end L24.end
  measures "d86" distance of L27.end L28.end
  measures "d188" distance between parallel lines of L28 L22
  measures "d189" distance between parallel lines of L28 L30
  measures "d190" distance between parallel lines of L26 L20
  measures "d191" distance between parallel lines of L26 L24
extrude "돌출11" cut sketch "스케치18" against normal blind 37
sketch "스케치20" plane through (78.1056, 5, 35) normal (0, 1, 0) x (1, 0, 0)
  line L0 (4.3978, -5) -> (-15.6022, -5) projected
  line L1 (-5.6022, -5) -> (-5.6022, 117.3008)
  arc A0 (-60.4557, 43.4791) -> (-60.4648, 26.5354) centre (-46.8872, 35) ccw projected
  line L2 (-46.8872, 35) -> (132.2335, 35)
  line L3 (9.3974, 7.5) -> (9.3974, 62.5) projected
  line L4 (31.3974, 23.5) -> (31.3974, 7.5) projected
  line L5 (-12.6022, 46) -> (-37.6022, 46)
  line L6 (-37.6022, 46) -> (-37.6022, 24)
  line L7 (-37.6022, 24) -> (-12.6022, 24)
  line L8 (-12.6022, 24) -> (-12.6022, 46)
  line L9 (-37.6022, 35) -> (-12.6022, 35) construction
  line L10 (-25.1022, 46) -> (-25.1022, 24) construction
  line L11 (31.3974, 23.5) -> (31.3974, 7.5) projected
  line L12 (31.3974, 7.5) -> (9.3974, 7.5) projected
  line L13 (9.3974, 7.5) -> (9.3974, 62.5) projected
  line L14 (9.3974, 62.5) -> (31.3974, 62.5) projected
  line L15 (31.3974, 62.5) -> (31.3974, 46.5) projected
  line L16 (31.3974, 46.5) -> (95.3291, 46.5) projected
  line L17 (95.3291, 46.5) -> (43.7484, 69.9799) projected
  line L18 (43.7484, 69.9799) -> (0, 69.9742) projected
  line L19 (0, 69.9742) -> (0, 0) projected
  line L20 (0, 0) -> (43.8605, 0) projected
  line L21 (43.8605, 0) -> (95.3771, 23.5) projected
  line L22 (95.3771, 23.5) -> (31.3974, 23.5) projected
  line L23 (44.8326, 74.9801) -> (116.6695, 42.2794) projected
  arc A1 (116.6752, 27.7198) -> (116.6695, 42.2794) centre (113.355, 34.9982) ccw projected
  line L24 (116.6752, 27.7198) -> (44.947, -5) projected
  line L25 (31.3974, 23.5) -> (31.3974, 7.5) projected
  line L26 (31.3974, 7.5) -> (9.3974, 7.5) projected
  line L27 (9.3974, 7.5) -> (9.3974, 62.5) projected
  line L28 (9.3974, 62.5) -> (31.3974, 62.5) projected
  line L29 (31.3974, 62.5) -> (31.3974, 46.5) projected
  line L30 (31.3974, 46.5) -> (95.3291, 46.5) projected
  line L31 (95.3291, 46.5) -> (43.7484, 69.9799) projected
  line L32 (43.7484, 69.9799) -> (0, 69.9742) projected
  line L33 (0, 69.9742) -> (0, 0) projected
  line L34 (0, 0) -> (43.8605, 0) projected
  line L35 (43.8605, 0) -> (95.3771, 23.5) projected
  line L36 (95.3771, 23.5) -> (31.3974, 23.5) projected
  line L37 (44.8326, 74.9801) -> (116.6695, 42.2794) projected
  arc A2 (116.6752, 27.7198) -> (116.6695, 42.2794) centre (113.355, 34.9982) ccw projected
  line L38 (116.6752, 27.7198) -> (44.947, -5) projected
  line L39 (270.2748, 35) -> (-184.3328, 35) projected
  arc A3 (-63.5629, 45.5989) -> (-63.5742, 24.4192) centre (-46.6022, 35) ccw projected
  line L40 (-63.5629, 45.5989) -> (-45.2097, 74.9682) projected
  line L41 (-45.2097, 74.9682) -> (44.8326, 74.9801) projected
  line L42 (44.947, -5) -> (-45.2335, -5) projected
  line L43 (-45.2335, -5) -> (-63.5742, 24.4192) projected
  line L44 (114.5979, 37.7287) -> (102.3974, 43.2825) projected
  line L45 (102.3974, 43.2825) -> (102.3974, 26.7024) projected
  line L46 (102.3974, 26.7024) -> (114.6001, 32.2688) projected
  arc A4 (114.6001, 32.2688) -> (114.5979, 37.7287) centre (113.355, 34.9982) ccw projected
  arc A5 (-63.5629, 45.5989) -> (-63.5742, 24.4192) centre (-46.6022, 35) ccw projected
  line L47 (-63.5629, 45.5989) -> (-45.2097, 74.9682) projected
  line L48 (-45.2097, 74.9682) -> (44.8326, 74.9801) projected
  line L49 (44.947, -5) -> (-45.2335, -5) projected
  line L50 (-45.2335, -5) -> (-63.5742, 24.4192) projected
  line L51 (114.5979, 37.7287) -> (102.3974, 43.2825) projected
  line L52 (102.3974, 43.2825) -> (102.3974, 26.7024) projected
  line L53 (102.3974, 26.7024) -> (114.6001, 32.2688) projected
  arc A6 (114.6001, 32.2688) -> (114.5979, 37.7287) centre (113.355, 34.9982) ccw projected
  point P0 (-78.1056, 35)
  point P1 (-25.1022, 35)
  point P2 (-29.2753, 35)
  point P3 (-25.1022, 35)
  dimension "d93" = 22
  dimension "d94" = 25
  dimension "d95" = 7
  constraints: 16 end point, 7 midpoint, 2 horizontal, 2 parallel, 2 point on line, 1 perpendicular, 1 vertical
  measures "d93" distance between parallel lines of L5 L7
  measures "d94" distance between parallel lines of L6 L8
  measures "d95" distance between parallel lines of L1 L8
extrude "돌출12" add sketch "스케치20" along normal blind 13 contours L8 L7 L6 L2 | L2 L6 L5 L8
sketch "스케치22" plane through (78.1056, 18, 35) normal (0, 1, 0) x (1, 0, 0)
  line L0 (-37.6022, 46) -> (-37.6022, 24) projected
  line L1 (-37.6022, 35) -> (-12.6022, 35)
  line L2 (-12.6022, 24) -> (-12.6022, 46) projected
  line L3 (-37.6022, 29) -> (-12.6022, 29)
  line L4 (-12.6022, 29) -> (-12.6022, 41)
  line L5 (-12.6022, 41) -> (-37.6022, 41)
  line L6 (-37.6022, 41) -> (-37.6022, 29)
  line L7 (-37.6022, 29) -> (-12.6022, 41) construction
  line L8 (-12.6022, 29) -> (-37.6022, 41) construction
  point P0 (-78.1056, 35)
  point P1 (-25.1022, 35)
  dimension "d98" = 12
  constraints: 14 end point, 5 midpoint, 2 parallel, 1 horizontal, 1 perpendicular, 1 point on line
  measures "d98" distance of L4.end L3.end
extrude "돌출13" cut sketch "스케치22" against normal blind 7
sketch "스케치23" plane through (87.503, 5, -27.5) normal (-1, 0, 0) x (0, 0, 1)
  line L0 (55, 12.5) -> (0, 12.5) projected
  line L1 (27.5, 12.5) -> (27.5, 17.5)
  line L2 (55, 17.5) -> (0, 17.5) projected
  line L3 (25, 17.5) -> (30, 17.5)
  line L4 (30, 17.5) -> (30, 12.5)
  line L5 (30, 12.5) -> (25, 12.5)
  line L6 (25, 12.5) -> (25, 17.5)
  line L7 (25, 17.5) -> (30, 12.5) construction
  line L8 (30, 17.5) -> (25, 12.5) construction
  point P0 (27.5, -5)
  point P1 (27.5, 15)
  dimension "d101" = 5
  constraints: 14 end point, 5 midpoint, 2 parallel, 1 horizontal, 1 perpendicular, 1 point on line
  measures "d101" distance of L4.end L5.end
extrude "돌출14" cut sketch "스케치23" against normal blind 24
sketch "스케치26" plane through (0, 0, 0) normal (0, 0, 1) x (1, 0, 0)
  line L0 (199.4606, 27.5719) -> (199.4606, 0) projected
  line L1 (123.0526, 0) -> (194.7808, 0) projected
  line L2 (199.4606, 0) -> (194.7751, 0) projected
  line L3 (199.4606, 0) -> (184.4606, 0)
  line L4 (184.4606, 0) -> (184.4606, -18.5052)
  arc A0 (184.4606, -11.5) -> (195.4606, -0.5) centre (184.4606, -0.5) ccw
  line L5 (184.4606, -0.5) -> (195.4606, -0.5)
  line L6 (195.4606, -0.5) -> (195.4606, 0)
  line L7 (195.4606, 0) -> (184.4606, 0)
  line L8 (184.4606, 0) -> (184.4606, -0.5)
  point P0 (0, 0)
  dimension "d113" = 15
  dimension "d114" = 22
  dimension "d115" = 0.5
  constraints: 12 end point, 4 point on line, 2 parallel, 2 point on circle, 1 centre point, 1 horizontal, 1 perpendicular, 1 vertical
  measures "d113" distance of L0.end L3.end
  measures "d114" diameter of A0
  measures "d115" distance from line of L1 L5.start
revolve "회전4" add sketch "스케치26" angle 360 about axis through (184.4606, 0, 0) along (0, -1, 0)
sketch "스케치27" plane through (0, 0, 0) normal (0, 0, 1) x (1, 0, 0)
  line L0 (173.4606, -0.5) -> (195.4606, -0.5) projected
  line L1 (173.4606, 0) -> (173.4606, -0.5) projected
  arc A0 (173.4606, -0.5) -> (195.4606, -0.5) centre (184.4606, -0.5) ccw projected
  line L2 (184.4606, -11.5) -> (184.4606, 13.9709)
  line L3 (184.4606, -11.5) -> (184.4606, -16.5195)
  arc A1 (184.4606, -13.1327) -> (184.4606, 2.8673) centre (184.4606, -5.1327) ccw
  point P0 (0, 0)
  constraints: 4 end point, 3 point on circle, 3 point on line, 2 vertical, 1 centre point
revolve "회전5" cut sketch "스케치27" angle 360 about axis through (184.4606, -11.5, 0) along (0, 1, 0) contours L2 A1 L0 | L0 A1 A0 L2 | A0 A1 L3
fillet "모깎기5" radius 0.5 1 edges at (177.4401, -8.9683, 0)
sketch "스케치28" plane through (0, 0, 0) normal (0, 0, 1) x (1, 0, 0)
  point P0 (0, 0)
sketch "스케치29" plane through (180.503, 5, 8.2976) normal (0, 1, 0) x (1, 0, 0)
  line L0 (0, 16.5801) -> (0, 0) projected
  line L1 (0, 0) -> (12.2027, 5.5664) projected
  arc A0 (12.2027, 5.5664) -> (12.2006, 11.0263) centre (10.9577, 8.2959) ccw projected
  line L2 (12.2006, 11.0263) -> (0, 16.5801) projected
  point P0 (-180.503, 8.2976)
extrude "돌출15" add sketch "스케치29" along normal blind 27.75
delete faces "면 삭제3" heal yes whole lump no faces at (184.5706, 32.75, 0.9154) (188.6381, 31.25, 4.5867)
ref_plane "작업 평면5" through (11.5034, 0, 0) normal (1, 0, 0) x (0, 1, 0)